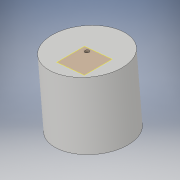
# Autodesk Inventor part: CylinderV02
Saved by Autodesk Inventor 2019.1 (Build 231200000, 200)
## iProperties
Created: 2018-11-04
Part Number: CylinderV02
Material: Generic
Document SubType Name: Modeling
Designer: steele
Density: 1 g/cm^3
Appearance: Default
Author: steele
Autodesk Inventor part; units mm, degrees
ref_plane "YZ Plane" through (0, 0, 0) normal (1, 0, 0) x (0, 1, 0)
ref_plane "XZ Plane" through (0, 0, 0) normal (0, 1, 0) x (-1, 0, 0)
ref_plane "XY Plane" through (0, 0, 0) normal (0, 0, 1) x (1, 0, 0)
ref_plane "Work Plane1" through (-29.2442, 7.9904, 7.7025) normal (-0.0927, 0.9957, 0) x (0.9957, 0.0927, 0)
sketch "Sketch3" plane through (-29.2442, 7.9904, 7.7025) normal (-0.0927, 0.9957, 0) x (0.9957, 0.0927, 0)
  circle A0 centre (-6, 8) radius 1.6815 projected
  circle A1 centre (-6, 8) radius 27.7483
  point P0 (28.3775, 7.7025)
  constraints: 1 centre point, 1 coincident
extrude "Extrusion3" add sketch "Sketch3" against normal blind 50.8
body "Solid1"
